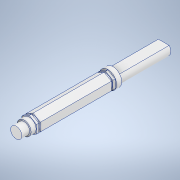
# Autodesk Inventor part: Axle1
Saved by Autodesk Inventor 2020.2 (Build 242310000, 310)
## iProperties
Created: 2020-01-19
Part Number: Axle1
Material: Aluminum 6061
Document SubType Name: Modeling
Designer: Paul Lefeuvre
Density: 2.7 g/cm^3
Appearance: Aluminum - Flat
Mass: 23.9891 g
Surface Area: 34.9021 cm^2
Volume: 8.88485 cm^3
Author: Paul Lefeuvre
Autodesk Inventor part; units mm, degrees
ref_plane "YZ Plane" through (0, 0, 0) normal (1, 0, 0) x (0, 1, 0)
sketch "Sketch1" plane through (0, 0, 0) normal (0, 0, 1) x (1, 0, 0)
  circle A0 centre (0, 0) radius 5.5
  circle A1 centre (0, 0) radius 7.5 construction
  line L0 (6.35, 3.6662) -> (6.35, -3.6662) construction
  line L1 (6.35, -3.6662) -> (0, -7.3323) construction
  line L2 (0, -7.3323) -> (-6.35, -3.6662) construction
  line L3 (-6.35, -3.6662) -> (-6.35, 3.6662) construction
  line L4 (-6.35, 3.6662) -> (0, 7.3323) construction
  line L5 (0, 7.3323) -> (6.35, 3.6662) construction
  line L6 (0, 0) -> (0, 12.7691) construction
  circle A2 centre (0, 0) radius 5 construction
  circle A3 centre (0, 0) radius 6.9
  circle A4 centre (0, 0) radius 4.4
  line L7 (0, 6.6395) -> (-5.75, 3.3198)
  line L8 (-5.75, 3.3198) -> (-5.75, -3.3198)
  line L9 (-5.75, -3.3198) -> (0, -6.6395)
  line L10 (0, -6.6395) -> (5.75, -3.3198)
  line L11 (5.75, -3.3198) -> (5.75, 3.3198)
  line L12 (5.75, 3.3198) -> (0, 6.6395)
  line L13 (4.2426, 3.5) -> (-4.2426, 3.5)
  dimension "d0" = 11
  dimension "d1" = 15
  dimension "d2" = 12.7
  dimension "d9" = 0.6
  dimension "d10" = 0.6
  dimension "d11" = 0.6
  dimension "d31" = 10
  dimension "d37" = 3.5
  constraints: 28 end point, 5 centre point, 4 coincident, 2 point on circle, 1 horizontal, 1 point on line, 1 vertical, 18 other
  measures "d0" diameter of A0
  measures "d1" diameter of A1
  measures "d2" distance of L0.start L3.end
  measures "d9" radial gap between concentric circles of A1 A3
  measures "d10" radial gap between concentric circles of A2 A4
  measures "d11" distance between parallel lines of L4 L7
  measures "d31" diameter of A2
  measures "d37" distance from line of point (0, 0) L13
extrude "Extrusion1" add sketch "Sketch1" along normal blind 4 contours A0 L13 A4 | L13 A4 A0 | L13 A4 | A4 L13 | A3 | L12 L11 L10 L9 L8 L7
extrude "Extrusion2" add sketch "Sketch1" along normal blind 66 contours A0 L13 A4 | L13 A4 A0 | L13 A4 | A4 L13 | L12 L11 L10 L9 L8 L7
extrude "Extrusion3" add sketch "Sketch1" along normal blind 70 contours A0 L13 A4 | L13 A4 A0 | L13 A4 | A4 L13
extrude "Extrusion4" add sketch "Sketch1" along normal blind 76.2 contours L13 A4 | A4 L13
extrude "Extrusion5" add sketch "Sketch1" against normal blind 40 contours A0 L13 A4 | A4 L13 picked at (5.0394, -0.7819) picked at (-0.9847, -1.0632)
ref_plane "Work Plane1" through (0, 0, 7) normal (0, 0, 1) x (1, 0, 0)
ref_plane "Work Plane2" through (0, 0, 63) normal (0, 0, 1) x (1, 0, 0)
sketch "Sketch2" plane through (0, 0, 7) normal (0, 0, 1) x (1, 0, 0)
  circle A0 centre (0, 0) radius 5.5
  circle A1 centre (0, 0) radius 7.5
  dimension "d23" = 11
  dimension "d24" = 2
  constraints: 2 centre point, 1 coincident
  measures "d23" diameter of A0
  measures "d24" radial gap between concentric circles of A0 A1
extrude "Extrusion6" cut sketch "Sketch2" against normal blind 1.2
sketch "Sketch3" plane through (5.75, -3.3198, 7) normal (0.5, -0.866, 0) x (0.866, 0.5, 0)
  point P0 (-3.3198, -7)
sketch "Sketch4" plane through (0, 0, 63) normal (0, 0, 1) x (1, 0, 0)
  circle A0 centre (0, 0) radius 5.5
  circle A1 centre (0, 0) radius 7.5
  dimension "d27" = 11
  dimension "d28" = 2
  constraints: 2 centre point, 1 coincident
  measures "d27" diameter of A0
  measures "d28" radial gap between concentric circles of A0 A1
extrude "Extrusion7" cut sketch "Sketch4" along normal blind 1.2
body "Solid1"
